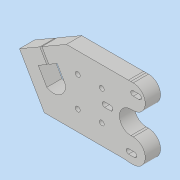
# Autodesk Inventor part: MMplate1
Saved by Autodesk Inventor 2017 (Build 210142000, 142)
## iProperties
Created: 2016-12-19
Part Number: MMplate1
Material: Generic
Document SubType Name: Modeling
Designer: Joshua Yuan
Density: 1 g/cm^3
Appearance: Default
Author: Joshua Yuan
Autodesk Inventor part; units mm, degrees
ref_plane "YZ Plane" through (0, 0, 0) normal (1, 0, 0) x (0, 1, 0)
ref_plane "XZ Plane" through (0, 0, 0) normal (0, 1, 0) x (-1, 0, 0)
ref_plane "XY Plane" through (0, 0, 0) normal (0, 0, 1) x (1, 0, 0)
sketch "Sketch1" plane through (0, 0, 0) normal (0, 0, 1) x (1, 0, 0)
  line L0 (40.2613, 48.6779) -> (47.3141, 52.7499)
  line L1 (56.0675, 57.8765) -> (63.1795, 45.5581)
  line L2 (40.2613, 48.6779) -> (47.3733, 36.3596)
  arc A0 (47.3733, 36.3596) -> (63.1795, 45.5581) centre (52.7696, 45.2664) ccw
  line L3 (24.6476, 52.8616) -> (41.5991, 62.6486)
  line L4 (63.7313, 75.4994) -> (115.2787, 75.4994)
  line L5 (24.6476, 52.8616) -> (45.3412, 17.0192)
  line L6 (45.3412, 17.0192) -> (112.2531, 17.0192)
  line L7 (-0.2016, 0) -> (173.7428, 0) projected
  line L8 (0, 4.7731) -> (0, 87.3731) projected
  line L9 (43.2997, 63.7032) -> (49.0147, 53.8045)
  line L10 (41.5991, 62.6486) -> (47.3141, 52.7499)
  line L11 (43.2997, 63.7032) -> (63.7313, 75.4994)
  line L12 (49.0147, 53.8045) -> (56.0675, 57.8765)
  circle A1 centre (117.3636, 46.0731) radius 29.5
  circle A2 centre (52.3236, 46.0731) radius 3.975 construction
  circle A3 centre (73.1795, 33.5731) radius 2.0193
  circle A4 centre (93.1795, 33.5731) radius 2.0193
  circle A5 centre (73.1795, 58.5731) radius 2.0193
  circle A6 centre (93.1795, 58.5731) radius 2.0193
  arc A7 (120.1894, 55.1693) -> (126.8661, 45.4194) centre (117.3636, 46.0731) ccw
  circle A8 centre (95.5267, 47.9836) radius 2
  circle A9 centre (119.2741, 67.91) radius 2
  circle A10 centre (139.2005, 44.1627) radius 2
  circle A11 centre (115.4531, 24.2362) radius 2
  line L13 (119.2741, 67.91) -> (115.4531, 24.2362) construction
  line L14 (139.2005, 44.1627) -> (95.5267, 47.9836) construction
  circle A12 centre (100.5267, 47.9836) radius 2
  circle A13 centre (124.2741, 67.91) radius 2
  circle A14 centre (120.4531, 24.2362) radius 2
  circle A15 centre (144.2005, 44.1627) radius 2
  circle A16 centre (119.3936, 46.0731) radius 29.5 construction
  circle A17 centre (119.3936, 46.0731) radius 9.525 construction
  line L15 (124.2741, 69.91) -> (119.2741, 69.91)
  line L16 (119.2741, 65.91) -> (124.2741, 65.91)
  line L17 (115.4531, 26.2362) -> (120.4531, 26.2362)
  line L18 (120.4531, 22.2362) -> (115.4531, 22.2362)
  line L19 (95.5267, 49.9836) -> (100.5267, 49.9836)
  line L20 (100.5267, 45.9836) -> (95.5267, 45.9836)
  line L21 (119.3936, 46.0731) -> (52.3236, 46.0731) construction
  circle A18 centre (97.5567, 47.9836) radius 2 construction
  circle A19 centre (121.3041, 67.91) radius 2 construction
  circle A20 centre (141.2305, 44.1627) radius 2 construction
  circle A21 centre (117.4831, 24.2362) radius 2 construction
  line L22 (139.2005, 46.1627) -> (144.2005, 46.1627)
  line L23 (144.2005, 42.1627) -> (139.2005, 42.1627)
  line L24 (141.2305, 44.1627) -> (97.5567, 47.9836) construction
  line L25 (121.3041, 67.91) -> (117.4831, 24.2362) construction
  line L26 (73.1795, 58.5731) -> (73.1795, 33.5731) construction
  line L27 (93.1795, 33.5731) -> (93.1795, 58.5731) construction
  arc A22 (119.3936, 55.5981) -> (119.3936, 75.5731) centre (119.3936, 65.5856) ccw
  arc A23 (119.3936, 16.5731) -> (119.3936, 36.5481) centre (119.3936, 26.5606) ccw
  line L28 (119.3936, 16.5731) -> (119.3936, 75.5731) construction
  line L29 (119.3936, 36.5481) -> (117.3636, 36.5481)
  line L30 (119.3936, 55.5981) -> (117.3636, 55.5981)
  line L31 (117.3636, 16.5731) -> (119.3936, 16.5731)
  line L32 (119.3936, 75.5731) -> (117.3636, 75.5731)
  arc A24 (126.8661, 45.4194) -> (120.1894, 55.1693) centre (117.3636, 46.0731) ccw construction
  point P0 (121.7741, 65.91)
  point P1 (117.3636, 46.0731)
  dimension "d8" = 18.288
  dimension "d9" = 14.224
  dimension "d10" = 10.414
  dimension "d13" = 11.43
  dimension "d14" = 11.43
  dimension "d15" = 2
  dimension "d17" = 59
  dimension "d18" = 7.95
  dimension "d19" = 9.144
  dimension "d20" = 9.2717
  dimension "d21" = 30
  dimension "d22" = 8.35
  dimension "d23" = 65.04
  dimension "d25" = 4.0386
  dimension "d26" = 4.0386
  dimension "d27" = 4.0386
  dimension "d28" = 4.0386
  dimension "d32" = 19.05
  dimension "d33" = 4
  dimension "d34" = 4
  dimension "d35" = 4
  dimension "d36" = 4
  dimension "d38" = 31
  dimension "d39" = 31
  dimension "d40" = 31
  dimension "d41" = 31
  dimension "d42" = 20
  dimension "d43" = 25
  dimension "d44" = 25
  dimension "d46" = 10
  dimension "d49" = 4
  dimension "d50" = 4
  dimension "d51" = 4
  dimension "d52" = 4
  dimension "d53" = 5
  dimension "d54" = 59
  dimension "d55" = 67.07
  dimension "d56" = 19.05
  dimension "d57" = 5
  dimension "d58" = 5
  dimension "d59" = 5
  dimension "d60" = 4
  dimension "d61" = 4
  dimension "d62" = 4
  dimension "d63" = 4
  dimension "d68" = 5
  dimension "d69" = 5
  dimension "d70" = 31
  dimension "d71" = 31
  dimension "d72" = 31
  dimension "d73" = 31
  constraints: 62 end point, 36 point on circle, 25 centre point, 16 tangent, 13 horizontal, 8 midpoint, 8 perpendicular, 6 point on line, 5 equal length, 5 parallel, 3 coincident, 3 vertical, 2 symmetric about line
  measures "d8" distance of L0.start L1.start
  measures "d9" distance of L0.start L2.end
  measures "d10" radius of A0
  measures "d13" distance between parallel lines of L5 L2
  measures "d14" distance of L9.start L9.end
  measures "d15" distance between parallel lines of L10 L9
  measures "d17" diameter of A1
  measures "d18" diameter of A2
  measures "d19" distance from line of L1 L21.end
  measures "d20" distance from line of L12 A0.centre
  measures "d21" angle of L7 L0
  measures "d22" distance from line of L12 L21.end
  measures "d23" distance of L21.end A1.centre
  measures "d25" diameter of A3
  measures "d26" diameter of A6
  measures "d27" diameter of A4
  measures "d28" diameter of A5
  measures "d32" diameter of A7
  measures "d33" diameter of A8
  measures "d34" diameter of A9
  measures "d35" diameter of A10
  measures "d36" diameter of A11
  measures "d38" distance of L14.start L13.end
  measures "d39" distance of L13.start L14.start
  measures "d40" distance of A8.centre L13.end
  measures "d41" distance of A8.centre L13.start
  measures "d42" distance of L26.start L27.end
  measures "d43" distance of L26.end L26.start
  measures "d44" distance of L27.start L27.end
  measures "d46" horizontal distance of L1.end L26.start
  measures "d49" diameter of A12
  measures "d50" diameter of A13
  measures "d51" diameter of A14
  measures "d52" diameter of A15
  measures "d53" distance of A8.centre A12.centre
  measures "d54" diameter of A16
  measures "d55" distance of L21.end A16.centre
  measures "d56" diameter of A17
  measures "d57" distance of L13.end A14.centre
  measures "d58" distance of A15.centre L14.start
  measures "d59" distance of L13.start A13.centre
  measures "d60" diameter of A18
  measures "d61" diameter of A19
  measures "d62" diameter of A20
  measures "d63" diameter of A21
  measures "d68" angle of L21 L24
  measures "d69" angle of L21 L14
  measures "d70" distance of L24.start L25.start
  measures "d71" distance of L25.end L24.start
  measures "d72" distance of L25.end L24.end
  measures "d73" distance of L24.end L25.start
extrude "Extrusion6" add sketch "Sketch1" along normal blind 12.7 contours L2 A0 L1 L12 L9 L11 L4 A1 L6 L5 L3 L10 L0 | A1 A22 L30 A7 L29 A23 | A1 A23 L31 | L32 A22 A1 picked at (102.6811, 61.1424)
body "Solid6"
